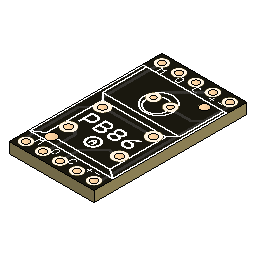
5631 PB86 Breakout (Autodesk Fusion 360 design; units mm, degrees)
part number: PB86_STEPSWITCH
Autodesk Fusion 360 part; units mm, degrees
sketch "sketch 306" plane through (0, 0, 0) normal (0, 0, 1) x (1, 0, 0)
  line L0 (-6.35, 11.43) -> (-6.35, -11.43)
  line L1 (-6.35, -11.43) -> (6.35, -11.43)
  line L2 (6.35, -11.43) -> (6.35, 11.43)
  line L3 (6.35, 11.43) -> (-6.35, 11.43)
extrude "Board" add sketch "sketch 306" along normal blind 1.57 makes body 1 in component "Board"
sketch "sketch 625" plane through (0, 0, 0) normal (0, 0, 1) x (1, 0, 0)
  line L0 (0.016, 0.016) -> (3.794, 0.016)
  line L1 (3.794, 0.016) -> (3.794, 3.794)
  line L2 (3.794, 3.794) -> (0.016, 3.794)
  line L3 (0.016, 3.794) -> (0.016, 0.016)
extrude "ADAFRUIT_3.5MM" add sketch "sketch 625" along normal blind 0.1 separate body makes body 2 in component "ADAFRUIT_3.5MM"
sketch "sketch 756" plane through (0, 0, 0) normal (0, 0, 1) x (1, 0, 0)
  line L0 (-6.2, -8.5) -> (6.2, -8.5)
  line L1 (6.2, -8.5) -> (6.2, 8.5)
  line L2 (6.2, 8.5) -> (-6.2, 8.5)
  line L3 (-6.2, 8.5) -> (-6.2, -8.5)
extrude "PB86" add sketch "sketch 756" along normal blind 0.1 separate body makes body 3 in component "PB86"
sketch "sketch 895" plane through (0, 0, 0) normal (0, 0, 1) x (1, 0, 0)
  line L0 (-6.35, -0.635) -> (5.58, -0.635)
  line L1 (5.58, -0.635) -> (5.58, 0.635)
  line L2 (5.58, 0.635) -> (-6.35, 0.635)
  line L3 (-6.35, 0.635) -> (-6.35, -0.635)
extrude "1X05_ROUND" add sketch "sketch 895" along normal blind 0.1 separate body makes body 4 in component "1X05_ROUND"
sketch "sketch 1026" plane through (0, 0, 0) normal (0, 0, 1) x (1, 0, 0)
  line L0 (-0.898, -0.898) -> (0.898, -0.898)
  line L1 (0.898, -0.898) -> (0.898, 0.898)
  line L2 (0.898, 0.898) -> (-0.898, 0.898)
  line L3 (-0.898, 0.898) -> (-0.898, -0.898)
extrude "PCBFEAT-REV-040" add sketch "sketch 1026" along normal blind 0.1 separate body makes body 5 in component "PCBFEAT-REV-040"
sketch "sketch 406" plane through (0, 0, 0) normal (0, 0, 1) x (1, 0, 0)
  circle A0 centre (-3.81, -7.625) radius 0.75
  circle A1 centre (3.81, 7.625) radius 0.65
  circle A2 centre (1.27, 5.08) radius 0.4
  circle A3 centre (-1.27, 5.08) radius 0.4
  circle A4 centre (-3.81, 0) radius 0.55
  circle A5 centre (3.81, 0) radius 0.55
  circle A6 centre (-3.81, -5.08) radius 0.55
  circle A7 centre (3.81, -5.08) radius 0.55
  circle A8 centre (-5.08, -10.16) radius 0.5
  circle A9 centre (-2.54, -10.16) radius 0.5
  circle A10 centre (0, -10.16) radius 0.5
  circle A11 centre (2.54, -10.16) radius 0.5
  circle A12 centre (5.08, -10.16) radius 0.5
  circle A13 centre (-5.08, 10.16) radius 0.5
  circle A14 centre (-2.54, 10.16) radius 0.5
  circle A15 centre (0, 10.16) radius 0.5
  circle A16 centre (2.54, 10.16) radius 0.5
  circle A17 centre (5.08, 10.16) radius 0.5
extrude "Extrude2" cut sketch "sketch 406" along normal blind 1.57 bodies 1 in component "Board"
component "Board" placed x (1, 0, 0) y (0, 1, 0) z (0, 0, 1) at (0, 0, 0)
component "ADAFRUIT_3.5MM" placed x (-1, 0, 0) y (0, 1, 0) z (0, 0, -1) at (1.524, -1.905, 0)
component "PB86" placed x (1, 0, 0) y (0, 1, 0) z (0, 0, 1) at (0, 0, 1.57)
component "1X05_ROUND" placed x (1, 0, 0) y (0, 1, 0) z (0, 0, 1) at (0, -10.16, 1.57)
component "1X05_ROUND" placed x (1, 0, 0) y (0, 1, 0) z (0, 0, 1) at (0, 10.16, 1.57)
component "PCBFEAT-REV-040" placed x (1, 0, 0) y (0, 1, 0) z (0, 0, 1) at (0, -5.207, 1.57)
named bodies: "Board", "ADAFRUIT_3.5MM", "PB86", "1X05_ROUND", "PCBFEAT-REV-040"
